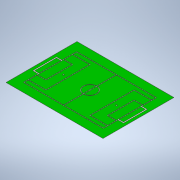
# Autodesk Inventor part: SoccerField_KidSize
Saved by Autodesk Inventor 2022 (Build 260153000, 153)
## iProperties
Created: 2022-10-30
Part Number: SoccerField_KidSize
Material: 一般
Document SubType Name: Modeling
Designer: Masato Kubotera
Density: 1 g/cm^3
Appearance: 既定
Author: Masato Kubotera
Autodesk Inventor part; units mm, degrees
ref_plane "YZ Plane" through (0, 0, 0) normal (1, 0, 0) x (0, 1, 0)
ref_plane "XZ Plane" through (0, 0, 0) normal (0, 1, 0) x (-1, 0, 0)
ref_plane "XY Plane" through (0, 0, 0) normal (0, 0, 1) x (1, 0, 0)
sketch "スケッチ1" plane through (0, 0, 0) normal (0, 0, 1) x (1, 0, 0)
  line L0 (-5500, -4025) -> (5500, -4025)
  line L1 (5500, -4025) -> (5500, 4025)
  line L2 (5500, 4025) -> (-5500, 4025)
  line L3 (-5500, 4025) -> (-5500, -4025)
  line L4 (-5500, -4025) -> (5500, 4025) construction
  line L5 (5500, -4025) -> (-5500, 4025) construction
  line L6 (5500, 0) -> (-5500, 0) construction
  line L7 (0, 4025) -> (0, -4025)
  line L8 (-4475, -2975) -> (4475, -2975)
  line L9 (4475, -2975) -> (4475, -2525)
  line L10 (4475, 2975) -> (-4475, 2975)
  line L11 (-4475, 2975) -> (-4475, -2975)
  line L12 (-4475, -2975) -> (4475, 2975) construction
  line L13 (4475, -2975) -> (-4475, 2975) construction
  line L14 (-4525, -3025) -> (4525, -3025)
  line L15 (4525, -3025) -> (4525, -1350)
  line L16 (4525, 3025) -> (-4525, 3025)
  line L17 (-4525, 3025) -> (-4525, -3025)
  line L18 (-4525, -3025) -> (4525, 3025) construction
  line L19 (4525, -3025) -> (-4525, 3025) construction
  line L20 (-4500, -3000) -> (4500, -3000) construction
  line L21 (4500, -3000) -> (4500, 3000) construction
  line L22 (4500, 3000) -> (-4500, 3000) construction
  line L23 (-4500, 3000) -> (-4500, -3000) construction
  line L24 (-4500, -3000) -> (4500, 3000) construction
  line L25 (4500, -3000) -> (-4500, 3000) construction
  line L26 (4500, 1300) -> (5100, 1300) construction
  line L27 (5100, 1300) -> (5100, -1300) construction
  line L28 (4525, 1250) -> (5050, 1250)
  line L29 (5050, 1250) -> (5050, -1250)
  line L30 (4525, 1350) -> (5050, 1350)
  line L31 (5150, 1350) -> (5150, -1350)
  line L32 (4500, -1300) -> (5100, -1300) construction
  line L33 (4525, -1250) -> (5050, -1250)
  line L34 (4525, -1350) -> (5150, -1350)
  line L35 (4500, 1500) -> (3500, 1500) construction
  line L36 (3500, 1500) -> (3500, -1500) construction
  line L37 (3500, -1500) -> (4500, -1500) construction
  line L38 (4475, 1525) -> (3475, 1525)
  line L39 (3475, 1525) -> (3475, -1525)
  line L40 (3475, -1525) -> (4475, -1525)
  line L41 (4475, -1475) -> (3525, -1475)
  line L42 (3525, -1475) -> (3525, 1475)
  line L43 (3525, 1475) -> (4475, 1475)
  line L44 (4500, 2500) -> (2500, 2500) construction
  line L45 (2500, 2500) -> (2500, -2500) construction
  line L46 (4475, 2525) -> (2475, 2525)
  line L47 (2475, 2525) -> (2475, -2525)
  line L48 (4475, 2475) -> (2525, 2475)
  line L49 (2525, 2475) -> (2525, -2475)
  line L50 (4475, -2525) -> (2475, -2525)
  line L51 (4475, -2475) -> (2525, -2475)
  line L52 (4500, -2500) -> (2500, -2500) construction
  arc A0 (25, 724.5688) -> (-25, 724.5688) centre (0, 0) ccw construction
  arc A1 (25, 774.5967) -> (-25, 774.5967) centre (0, 0) ccw construction
  circle A2 centre (0, 0) radius 750 construction
  line L53 (25, 2975) -> (25, 774.5967)
  line L54 (-25, 2975) -> (-25, 774.5967)
  line L55 (-75, 25) -> (-25, 25)
  line L56 (75, 25) -> (75, -25)
  line L57 (75, -25) -> (25, -25)
  line L58 (-75, -25) -> (-75, 25)
  line L59 (-75, 25) -> (75, -25) construction
  line L60 (75, 25) -> (-75, -25) construction
  line L61 (2925, 25) -> (2975, 25)
  line L62 (3075, 25) -> (3075, -25)
  line L63 (3075, -25) -> (3025, -25)
  line L64 (2925, -25) -> (2925, 25)
  line L65 (2925, 25) -> (3075, -25) construction
  line L66 (3075, 25) -> (2925, -25) construction
  line L67 (2975, 75) -> (3025, 75)
  line L68 (3025, 75) -> (3025, 25)
  line L69 (3025, -75) -> (2975, -75)
  line L70 (2975, -75) -> (2975, -25)
  line L71 (2975, 75) -> (3025, -75) construction
  line L72 (3025, 75) -> (2975, -75) construction
  line L73 (4475, 2475) -> (4475, 2525) construction
  line L74 (4475, 2525) -> (4475, 2975)
  line L75 (4475, 1475) -> (4475, 1525) construction
  line L76 (4475, 1525) -> (4475, 2475)
  line L77 (4525, 1250) -> (4525, 1350) construction
  line L78 (5050, 1350) -> (5150, 1350)
  line L79 (4525, 1350) -> (4525, 3025)
  line L80 (4525, -1250) -> (4525, 1250)
  line L81 (4525, -1350) -> (4525, -1250) construction
  line L82 (4475, -1525) -> (4475, -1475) construction
  line L83 (4475, -1475) -> (4475, 1475)
  line L84 (4475, -2525) -> (4475, -2475) construction
  line L85 (4475, -2475) -> (4475, -1525)
  line L86 (2975, -25) -> (2975, 25) construction
  line L87 (2975, 25) -> (3025, 25) construction
  line L88 (3025, 25) -> (3025, -25) construction
  line L89 (3025, -25) -> (3025, -75)
  line L90 (3025, 25) -> (3075, 25)
  line L91 (2975, -25) -> (2925, -25)
  line L92 (2975, 25) -> (2975, 75)
  line L93 (3025, -25) -> (2975, -25) construction
  arc A3 (585.0661, 428.162) -> (25, 724.5688) centre (0, 0) ccw
  arc A4 (625.4155, 457.6904) -> (25, 774.5967) centre (0, 0) ccw
  line L94 (25, 724.5688) -> (25, 25)
  line L95 (25, 774.5967) -> (25, 724.5688) construction
  line L96 (-25, 724.5688) -> (-25, 25)
  arc A5 (-25, 774.5967) -> (-25, -774.5967) centre (0, 0) ccw
  line L97 (-25, 774.5967) -> (-25, 724.5688) construction
  line L98 (-25, 25) -> (-25, -25) construction
  arc A6 (-25, 724.5688) -> (-25, -724.5688) centre (0, 0) ccw
  line L99 (25, -724.5688) -> (25, -774.5967) construction
  arc A7 (-25, -724.5688) -> (25, -724.5688) centre (0, 0) ccw construction
  arc A8 (-25, -774.5967) -> (25, -774.5967) centre (0, 0) ccw construction
  arc A9 (25, -774.5967) -> (625.4155, 457.6904) centre (0, 0) ccw
  line L100 (25, -774.5967) -> (25, -2975)
  line L101 (-25, -774.5967) -> (-25, -2975)
  line L102 (-25, -724.5688) -> (-25, -774.5967) construction
  arc A10 (25, -724.5688) -> (585.0661, 428.162) centre (0, 0) ccw
  line L103 (-25, 25) -> (0, 25) construction
  line L104 (0, 25) -> (25, 25) construction
  line L105 (25, 25) -> (25, -25) construction
  line L106 (25, 25) -> (75, 25)
  line L107 (25, -25) -> (-25, -25) construction
  line L108 (25, -25) -> (25, -724.5688)
  line L109 (-25, -25) -> (-25, -724.5688)
  line L110 (-25, -25) -> (-75, -25)
  point P0 (3000, 0)
  point P1 (452.5, -127.5)
  point P2 (447.5, -247.5)
  point P3 (302.5, -2.5)
  point P4 (297.5, -2.5)
  point P5 (297.5, 2.5)
  point P6 (302.5, 2.5)
  point P7 (2.5, 77.4597)
  point P8 (2.5, -77.4597)
  point P9 (447.5, -252.5)
  point P10 (2.5, -2.5)
  point P11 (25, 724.5688)
  point P12 (2.5, 72.4569)
  point P13 (2.5, 2.5)
  point P14 (-2.5, 2.5)
  point P15 (-2.5, 72.4569)
  point P16 (-25, 724.5688)
  point P17 (-2.5, -2.5)
  point P18 (-2.5, 77.4597)
  point P19 (-2.5, 77.4597)
  point P20 (452.5, -132.5)
  point P21 (0, 3025)
  point P22 (0, -3025)
  dimension "d1" = 1000
  dimension "d2" = 50
  dimension "d3" = 50
  dimension "d4" = 1000
  dimension "d5" = 6000
  dimension "d6" = 9000
  dimension "d7" = 2600
  dimension "d8" = 100
  dimension "d9" = 100
  dimension "d10" = 600
  dimension "d11" = 50
  dimension "d12" = 50
  dimension "d13" = 3000
  dimension "d14" = 1000
  dimension "d15" = 50
  dimension "d16" = 50
  dimension "d17" = 2000
  dimension "d18" = 5000
  dimension "d19" = 1500
  dimension "d20" = 50
  dimension "d21" = 1450
  dimension "d22" = 50
  dimension "d23" = 50
  dimension "d24" = 150
  dimension "d25" = 50
  dimension "d26" = 50
  dimension "d27" = 150
  dimension "d28" = 150
  dimension "d29" = 1500
  constraints: 222 end point, 84 perpendicular, 56 parallel, 21 point on circle, 18 midpoint, 17 point on line, 16 horizontal, 12 symmetric about line, 11 centre point, 3 coincident, 12 other
  measures "d1" distance between parallel lines of L1 L21
  measures "d2" distance between parallel lines of L9 L15
  measures "d3" distance between parallel lines of L16 L10
  measures "d4" distance between parallel lines of L2 L16
  measures "d5" distance of L20.end L21.end
  measures "d6" distance of L21.end L22.end
  measures "d7" distance between parallel lines of L32 L26
  measures "d8" distance between parallel lines of L29 L31
  measures "d9" distance between parallel lines of L30 L28
  measures "d10" distance between parallel lines of L21 L27
  measures "d11" distance between parallel lines of L38 L43
  measures "d12" distance between parallel lines of L39 L42
  measures "d13" distance between parallel lines of L37 L35
  measures "d14" distance between parallel lines of L21 L36
  measures "d15" distance between parallel lines of L48 L46
  measures "d16" distance between parallel lines of L47 L49
  measures "d17" distance between parallel lines of L45 L21
  measures "d18" distance of L44.end L45.end
  measures "d19" diameter of A2
  measures "d20" radial gap between concentric circles of A1 A0
  measures "d21" diameter of A0
  measures "d22" distance between parallel lines of L54 L53
  measures "d23" distance of L56.start L56.end
  measures "d24" distance of L56.end L58.start
  measures "d25" distance of L62.start L62.end
  measures "d26" distance of L69.start L69.end
  measures "d27" distance of L62.end L64.start
  measures "d28" distance of L69.end L67.start
  measures "d29" distance from line of L21 point (3000, 0)
extrude "押し出し1" add sketch "スケッチ1" along normal blind 3 contours L7 L14 L15 L34 L31 L78 L30 L79 L16 L2 L1 L0 | L100 A9 A4 L53 L10 L74 L46 L47 L50 L9 L8 | L28 L29 L33 L80 | L38 L39 L40 L85 L51 L49 L48 L76 | L41 L42 L43 L83 | L106 L94 A3 A10 L108 L57 L56
extrude "押し出し2" add sketch "スケッチ1" along normal blind 3 separate body contours L7 L8 L9 L50 L47 L46 L74 L10 L16 L79 L30 L78 L31 L34 L15 L14 | L7 L10 L53 A4 A9 L100 L8 | L61 L92 L67 L68 L90 L62 L63 L89 L69 L70 L91 L64
mirror "ミラー1" about plane through (0, 0, 0) normal (1, 0, 0) bodies 2 1
equation "\"d3\" = d2"
equation "\"d4\" = d1"
equation "\"d11\" = d2"
equation "\"d12\" = d2"
equation "\"d15\" = d2"
equation "\"d16\" = d2"
equation "\"d20\" = d2"
equation "\"d21\" = d19 - d20"
equation "\"d22\" = d2"
equation "\"d23\" = d2"
equation "\"d24\" = 3 * d23"
equation "\"d25\" = d2"
equation "\"d26\" = d2"
equation "\"d27\" = d24"
equation "\"d28\" = d24"
